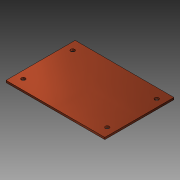
# Autodesk Inventor part: Copper_Plate
Saved by Autodesk Inventor 2018 (Build 220112000, 112)
## iProperties
Created: 2017-06-02
Part Number: Copper_Plate
Material: Copper
Document SubType Name: Modeling
Designer: AYUSH SHUKLA
Density: 8.94 g/cm^3
Appearance: Copper - Satin
Author: AYUSH SHUKLA
Autodesk Inventor part; units mm, degrees
ref_plane "YZ Plane" through (0, 0, 0) normal (1, 0, 0) x (0, 1, 0)
ref_plane "XZ Plane" through (0, 0, 0) normal (0, 1, 0) x (-1, 0, 0)
ref_plane "XY Plane" through (0, 0, 0) normal (0, 0, 1) x (1, 0, 0)
sketch "Sketch1" plane through (0, 0, 0) normal (0, 0, 1) x (1, 0, 0)
  circle A0 centre (7.5, -10) radius 2 projected
  circle A1 centre (7.5, -60) radius 2 projected
  line L0 (0, 0) -> (0, -69.9999) projected
  line L1 (0, -69.9999) -> (15, -69.9999) projected
  line L2 (15, 0) -> (15, -69.9999) projected
  line L3 (0, 0) -> (15, 0) projected
  line L4 (15, 0) -> (-85, 0)
  line L5 (-85, 0) -> (-85, -70)
  line L6 (-85, -70) -> (15, -70)
  line L7 (15, -70) -> (15, 0)
  circle A2 centre (-77.5, -10) radius 2 projected
  circle A3 centre (-77.5, -60) radius 2 projected
  line L8 (-85, 0) -> (-85, -69.9999) projected
  line L9 (-85, -69.9999) -> (-70, -69.9999) projected
  line L10 (-70, 0) -> (-70, -69.9999) projected
  line L11 (-85, 0) -> (-70, 0) projected
  dimension "d0" = 100
  dimension "d1" = 70
  constraints: 8 end point, 2 parallel, 1 horizontal, 1 perpendicular
  measures "d0" distance of L6.end L5.end
  measures "d1" distance of L5.end L4.end
extrude "Extrusion1" add sketch "Sketch1" along normal blind 2
body "Solid1"
